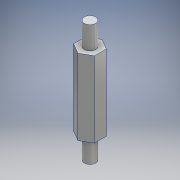
# Autodesk Inventor part: スペーサー　両雄ねじ　m3-20
Saved by Autodesk Inventor 2016 (Build 200138000, 138)
## iProperties
Created: 2016-03-06
Part Number: スペーサー　両雄ねじ　m3-20
Material: アルミニウム 2014-T4
Document SubType Name: Modeling
Designer: Takumi
Density: 2.8 g/cm^3
Appearance: アルミニウム - フラット
Mass: 1.70455 g
Surface Area: 5.46543 cm^2
Volume: 0.608768 cm^3
Author: Takumi
Autodesk Inventor part; units mm, degrees
ref_plane "YZ Plane" through (0, 0, 0) normal (1, 0, 0) x (0, 1, 0)
ref_plane "XZ Plane" through (0, 0, 0) normal (0, 1, 0) x (-1, 0, 0)
ref_plane "XY Plane" through (0, 0, 0) normal (0, 0, 1) x (1, 0, 0)
sketch "スケッチ1" plane through (0, 0, 0) normal (0, 0, 1) x (1, 0, 0)
  line L0 (-2.75, 1.5877) -> (0, 3.1754)
  line L1 (0, 3.1754) -> (2.75, 1.5877)
  line L2 (2.75, 1.5877) -> (2.75, -1.5877)
  line L3 (2.75, -1.5877) -> (0, -3.1754)
  line L4 (0, -3.1754) -> (-2.75, -1.5877)
  line L5 (-2.75, -1.5877) -> (-2.75, 1.5877)
  circle A0 centre (0, 0) radius 1.5
  dimension "d0" = 5.5
  dimension "d1" = 3
  constraints: 12 end point, 2 coincident, 1 centre point, 1 vertical, 13 other
  measures "d0" distance of L1.end L0.start
  measures "d1" diameter of A0
extrude "押し出し1" add sketch "スケッチ1" along normal blind 20 contours L0 L1 L2 L3 L4 L5 | A0
sketch "スケッチ2" plane through (0, 0, 20) normal (0, 0, 1) x (1, 0, 0)
  circle A0 centre (0, 0) radius 1.5
  dimension "d4" = 3
  constraints: 1 centre point, 1 coincident
  measures "d4" diameter of A0
extrude "押し出し2" add sketch "スケッチ2" along normal blind 6
extrude "押し出し3" add sketch "スケッチ1" against normal blind 6 contours A0
